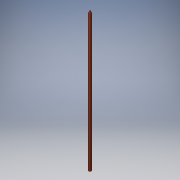
# Autodesk Inventor part: haste_para_raio
Saved by Autodesk Inventor 2019.4 (Build 234330000, 330)
## iProperties
Created: 2021-02-17
Part Number: haste_para_raio
Material: Cobre
Document SubType Name: Modeling
Designer: Lattes
Density: 8.94 g/cm^3
Appearance: Cobre - Acetinado
Author: Lattes
Autodesk Inventor part; units mm, degrees
ref_plane "YZ Plane" through (0, 0, 0) normal (1, 0, 0) x (0, 1, 0)
ref_plane "XZ Plane" through (0, 0, 0) normal (0, 1, 0) x (-1, 0, 0)
ref_plane "XY Plane" through (0, 0, 0) normal (0, 0, 1) x (1, 0, 0)
sketch "Esboço2" plane through (0, 0, 0) normal (0, 0, 1) x (1, 0, 0)
  line L0 (0, 0) -> (5, 0)
  line L1 (5, 0) -> (5, 500)
  line L2 (5, 500) -> (0, 510.7225)
  line L3 (5, 500) -> (16.831, 500) construction
  line L4 (0, 0) -> (0, 17.6655)
  line L5 (0, 510.7225) -> (0, 0)
  dimension "d1" = 5
  dimension "d2" = 500
  dimension "d3" = 115
  constraints: 12 end point, 2 horizontal, 1 collinear, 1 equal length, 1 perpendicular, 1 vertical
  measures "d1" distance of L0.start L0.end
  measures "d2" distance of L0.end L1.end
  measures "d3" angle of L3 L2
revolve "Revolução1" add sketch "Esboço2" angle 360 about axis through (0, 0, 0) along (0, 1, 0)
